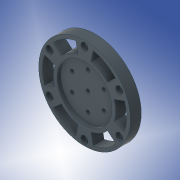
# Autodesk Inventor part: SJ002
Saved by Autodesk Inventor 2017 SP1 (Build 210196100, 196)
## iProperties
Created: 2017-06-01
Part Number: SJ002
Material: ABS Plastic
Document SubType Name: Modeling
Designer: Zach
Density: 1.06 g/cm^3
Appearance: CR Dark Blue
Author: Zach
Autodesk Inventor part; units mm, degrees
ref_plane "YZ Plane" through (0, 0, 0) normal (1, 0, 0) x (0, 1, 0)
ref_plane "XZ Plane" through (0, 0, 0) normal (0, 1, 0) x (-1, 0, 0)
ref_plane "XY Plane" through (0, 0, 0) normal (0, 0, 1) x (1, 0, 0)
sketch "Sketch2" plane through (0, 0, 0) normal (0, 0, 1) x (1, 0, 0)
  circle A0 centre (0, 0) radius 62.5
  circle A1 centre (0, 0) radius 2.5
  dimension "d0" = 125
  dimension "d1" = 5
  constraints: 2 centre point, 2 coincident
  measures "d0" diameter of A0
  measures "d1" diameter of A1
extrude "Extrusion1" add sketch "Sketch2" along normal blind 15
sketch "Sketch4" plane through (0, 0, 0) normal (0, 0, -1) x (-1, 0, 0)
  circle A0 centre (0, 25) radius 2.575
  circle A1 centre (-21.6506, 12.5) radius 2.575
  circle A2 centre (-21.6506, -12.5) radius 2.575
  circle A3 centre (0, -25) radius 2.575
  circle A4 centre (21.6506, -12.5) radius 2.575
  circle A5 centre (21.6506, 12.5) radius 2.575
  point P0 (0, 0)
  dimension "d8" = 5.15
  dimension "d9" = 25
  dimension "d12" = 360
  constraints: 6 centre point, 1 vertical alignment, 13 other
  measures "d8" diameter of A0
  measures "d9" distance of point (0, 0) A0.centre
extrude "Extrusion3" cut sketch "Sketch4" against normal through all
sketch "Sketch5" plane through (0, 0, 15) normal (0, 0, 1) x (1, 0, 0)
  circle A0 centre (0, 0) radius 37.5
  dimension "d16" = 75
  constraints: 1 centre point, 1 coincident
  measures "d16" diameter of A0
extrude "Extrusion4" cut sketch "Sketch5" against normal blind 5
sketch "Sketch6" plane through (0, 0, 15) normal (0, 0, 1) x (1, 0, 0)
  circle A0 centre (0, 55) radius 2.5
  circle A1 centre (-47.6314, 27.5) radius 2.5
  circle A2 centre (-47.6314, -27.5) radius 2.5
  circle A3 centre (0, -55) radius 2.5
  circle A4 centre (47.6314, -27.5) radius 2.5
  circle A5 centre (47.6314, 27.5) radius 2.5
  point P0 (0, 0)
  dimension "d19" = 5
  dimension "d20" = 55
  dimension "d23" = 360
  constraints: 6 centre point, 13 other
  measures "d19" diameter of A0
  measures "d20" distance of point (0, 0) A0.centre
extrude "Extrusion5" cut sketch "Sketch6" against normal through all
sketch "Sketch8" plane through (0, 0, 15) normal (0, 0, 1) x (1, 0, 0)
  circle A0 centre (0, 0) radius 37.5 projected
  circle A1 centre (0, 0) radius 62.5 projected
  circle A2 centre (0, 55) radius 2.5 projected
  circle A3 centre (0, 55) radius 5
  circle A4 centre (-47.6314, 27.5) radius 5
  circle A5 centre (-47.6314, -27.5) radius 5
  circle A6 centre (0, -55) radius 5
  circle A7 centre (47.6314, -27.5) radius 5
  circle A8 centre (47.6314, 27.5) radius 5
  point P0 (-56.2917, 32.5)
  point P1 (-56.2917, -32.5)
  point P2 (0, -65)
  point P3 (56.2917, -32.5)
  point P4 (56.2917, 32.5)
  dimension "d28" = 10
  dimension "d31" = 360
  constraints: 6 centre point, 1 coincident, 17 other
  measures "d28" diameter of A3
extrude "Extrusion6" cut sketch "Sketch8" against normal blind 5 contours A2 | A3 | A4 | A5 | A6 | A7 | A8
sketch "Sketch9" plane through (0, 0, 15) normal (0, 0, 1) x (1, 0, 0)
  circle A0 centre (0, 0) radius 2.5 construction
  circle A1 centre (0, 0) radius 42.5 construction
  circle A2 centre (0, 0) radius 57.5 construction
  line L0 (40.4629, 13) -> (54.61, 18)
  line L1 (40.4629, -13) -> (54.61, -18)
  line L2 (0, 0) -> (92.9665, 0) construction
  arc A3 (40.4629, -13) -> (40.4629, 13) centre (0, 0) ccw
  arc A4 (54.61, -18) -> (54.61, 18) centre (0, 0) ccw
  circle A5 centre (0, 0) radius 42.5 construction
  line L3 (8.9731, 41.5419) -> (11.7165, 56.2936)
  arc A6 (31.4898, 28.5419) -> (8.9731, 41.5419) centre (0, 0) ccw
  line L4 (31.4898, 28.5419) -> (42.8934, 38.2936)
  circle A7 centre (0, 0) radius 57.5 construction
  arc A8 (42.8934, 38.2936) -> (11.7165, 56.2936) centre (0, 0) ccw
  circle A9 centre (0, 0) radius 42.5 construction
  line L5 (-31.4898, 28.5419) -> (-42.8934, 38.2936)
  arc A10 (-8.9731, 41.5419) -> (-31.4898, 28.5419) centre (0, 0) ccw
  line L6 (-8.9731, 41.5419) -> (-11.7165, 56.2936)
  circle A11 centre (0, 0) radius 57.5 construction
  arc A12 (-11.7165, 56.2936) -> (-42.8934, 38.2936) centre (0, 0) ccw
  circle A13 centre (0, 0) radius 42.5 construction
  line L7 (-40.4629, -13) -> (-54.61, -18)
  arc A14 (-40.4629, 13) -> (-40.4629, -13) centre (0, 0) ccw
  line L8 (-40.4629, 13) -> (-54.61, 18)
  circle A15 centre (0, 0) radius 57.5 construction
  arc A16 (-54.61, 18) -> (-54.61, -18) centre (0, 0) ccw
  circle A17 centre (0, 0) radius 42.5 construction
  line L9 (-8.9731, -41.5419) -> (-11.7165, -56.2936)
  arc A18 (-31.4898, -28.5419) -> (-8.9731, -41.5419) centre (0, 0) ccw
  line L10 (-31.4898, -28.5419) -> (-42.8934, -38.2936)
  circle A19 centre (0, 0) radius 57.5 construction
  arc A20 (-42.8934, -38.2936) -> (-11.7165, -56.2936) centre (0, 0) ccw
  circle A21 centre (0, 0) radius 42.5 construction
  line L11 (31.4898, -28.5419) -> (42.8934, -38.2936)
  arc A22 (8.9731, -41.5419) -> (31.4898, -28.5419) centre (0, 0) ccw
  line L12 (8.9731, -41.5419) -> (11.7165, -56.2936)
  circle A23 centre (0, 0) radius 57.5 construction
  arc A24 (11.7165, -56.2936) -> (42.8934, -38.2936) centre (0, 0) ccw
  dimension "d35" = 85
  dimension "d36" = 115
  dimension "d37" = 13
  dimension "d38" = 18
  dimension "d41" = 360
  constraints: 48 point on circle, 26 end point, 24 centre point, 12 concentric, 7 coincident, 1 horizontal, 86 other
  measures "d35" diameter of A1
  measures "d36" diameter of A2
  measures "d37" vertical distance of L0.start point (0, 0)
  measures "d38" vertical distance of L0.end point (0, 0)
extrude "Extrusion7" cut sketch "Sketch9" against normal through all
body "Solid1"
